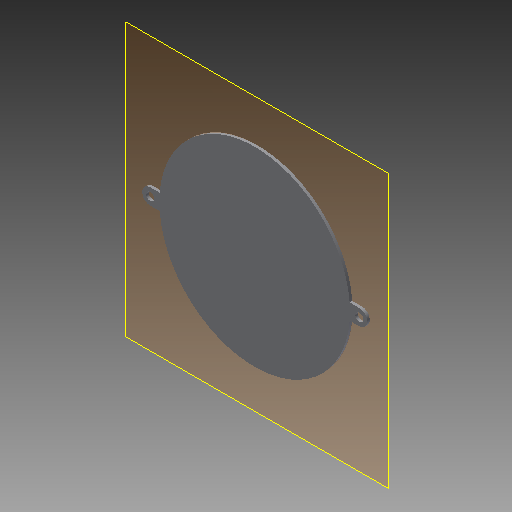
# Autodesk Inventor part: frame4
Saved by Autodesk Inventor 2017 (Build 210142000, 142)
## iProperties
Created: 2016-10-18
Part Number: frame4
Material: Generic
Document SubType Name: Modeling
Designer: Paulo Loma
Density: 1 g/cm^3
Appearance: Default
Author: Paulo Loma
Autodesk Inventor part; units mm, degrees
ref_plane "YZ Plane" through (0, 0, 0) normal (1, 0, 0) x (0, 1, 0)
ref_plane "XZ Plane" through (0, 0, 0) normal (0, 1, 0) x (-1, 0, 0)
ref_plane "XY Plane" through (0, 0, 0) normal (0, 0, 1) x (1, 0, 0)
ref_plane "Work Plane1" through (0, 0, 5) normal (0, 0, 1) x (1, 0, 0)
sketch "Sketch1" plane through (0, 0, 5) normal (0, 0, 1) x (1, 0, 0)
  circle A0 centre (-39.5, 0) radius 1.5
  arc A1 (-39.5, 3) -> (-39.5, -3) centre (-39.5, 0) ccw
  line L0 (-39.5, -3) -> (-35.8748, -3)
  line L1 (-39.5, 3) -> (-35.8748, 3)
  circle A2 centre (39.5, 0) radius 1.5
  arc A3 (39.5, -3) -> (39.5, 3) centre (39.5, 0) ccw
  line L2 (39.5, -3) -> (35.8748, -3)
  line L3 (39.5, 3) -> (35.8748, 3)
  arc A4 (-35.8748, -3) -> (35.8748, -3) centre (0, 0) ccw
  arc A5 (35.8748, 3) -> (-35.8748, 3) centre (0, 0) ccw
  constraints: 8 end point, 8 point on circle, 6 centre point, 3 horizontal, 2 coincident, 2 tangent, 1 parallel
extrude "Extrusion3" add sketch "Sketch1" along normal blind 1
body "Solid3"
